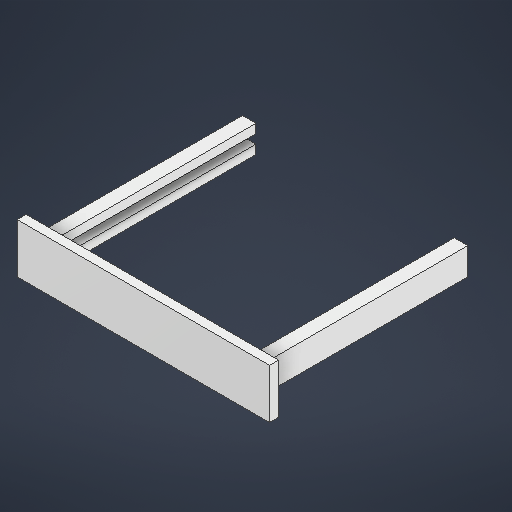
# Autodesk Inventor part: clip_pcb-command
Saved by Autodesk Inventor 2025.4 (Build 294407000, 407)
## iProperties
Created: 2025-12-22
Part Number: clip_pcb-command
Material: ABS Plastic
Document SubType Name: Modeling
Designer: sam
Density: 1.06 g/cm^3
Appearance: Smooth - White
Author: sam
Autodesk Inventor part; units mm, degrees
ref_plane "YZ Plane" through (0, 0, 0) normal (1, 0, 0) x (0, 1, 0)
ref_plane "XZ Plane" through (0, 0, 0) normal (0, 1, 0) x (-1, 0, 0)
ref_plane "XY Plane" through (0, 0, 0) normal (0, 0, 1) x (1, 0, 0)
sketch "Sketch1" plane through (0, 0, 0) normal (0, 1, 0) x (-1, 0, 0)
  line L0 (-25, -25) -> (25, -25)
  line L1 (25, -25) -> (25, 25)
  line L2 (25, 25) -> (-25, 25)
  line L3 (-25, 25) -> (-25, -25)
  line L4 (-25, -25) -> (25, 25) construction
  line L5 (25, -25) -> (-25, 25) construction
  line L6 (25, 21) -> (-25, 21)
  line L7 (22, 21) -> (22, -25)
  line L8 (-22, 21) -> (-22, -25)
  point P0 (0, 0)
  dimension "d0" = 50
  dimension "d1" = 50
  dimension "d2" = 4
  dimension "d3" = 3
  dimension "d4" = 3
  constraints: 18 end point, 6 point on line, 4 perpendicular, 2 midpoint, 2 parallel, 1 horizontal
  measures "d0" distance of L2.end L1.end
  measures "d1" distance of L1.end L0.end
  measures "d2" distance between parallel lines of L2 L6
  measures "d3" distance between parallel lines of L3 L8
  measures "d4" distance between parallel lines of L1 L7
extrude "Extrusion1" add sketch "Sketch1" along normal blind 2 contours L3 L6 L8 L0 | L3 L2 L1 L6 | L7 L6 L1 L0
sketch "Sketch2" plane through (0, 2, 0) normal (0, 1, 0) x (1, 0, 0)
  line L0 (-22, 25) -> (-25, 25) projected
  line L1 (-25, 25) -> (-25, -25) projected
  line L2 (-25, -25) -> (25, -25) projected
  line L3 (25, -25) -> (25, 25) projected
  line L4 (25, 25) -> (22, 25) projected
  line L5 (22, 25) -> (22, -21) projected
  line L6 (22, -21) -> (-22, -21) projected
  line L7 (-22, -21) -> (-22, 25) projected
  line L8 (-25, -25) -> (25, -25)
  line L9 (25, -25) -> (25, -23)
  line L10 (25, -23) -> (-25, -23)
  line L11 (-25, -23) -> (-25, -25)
  point P0 (0, 0)
  dimension "d7" = 2
  constraints: 8 end point, 2 parallel, 1 horizontal, 1 perpendicular, 1 point on line
  measures "d7" distance of L9.end L8.end
extrude "Extrusion2" add sketch "Sketch2" along normal blind 9 contours L10 L3 L2 L1
sketch "Sketch3" plane through (0, 2, 0) normal (0, 1, 0) x (1, 0, 0)
  line L0 (-25, -23) -> (25, -23) projected
  line L1 (25, -23) -> (25, 25) projected
  line L2 (25, 25) -> (22, 25) projected
  line L3 (22, 25) -> (22, -21) projected
  line L4 (22, -21) -> (-22, -21) projected
  line L5 (-22, -21) -> (-22, 25) projected
  line L6 (-22, 25) -> (-25, 25) projected
  line L7 (-25, 25) -> (-25, -23) projected
  line L8 (-25, -23) -> (-24.2, -23)
  line L9 (-24.2, -23) -> (-24.2, 25)
  line L10 (-24.2, 25) -> (-25, 25)
  line L11 (-25, 25) -> (-25, -23)
  line L12 (25, -23) -> (24.2, -23)
  line L13 (24.2, -23) -> (24.2, 25)
  line L14 (24.2, 25) -> (25, 25)
  line L15 (25, 25) -> (25, -23)
  point P0 (0, 0)
  dimension "d10" = 0.8
  dimension "d11" = 0.8
  constraints: 16 end point, 4 parallel, 2 horizontal, 2 perpendicular, 2 point on line
  measures "d10" distance of L10.end L9.end
  measures "d11" distance of L13.end L14.end
extrude "Extrusion3" add sketch "Sketch3" along normal blind 2 contours L7 L6 L9 L0 | L13 L2 L1 L0
sketch "Sketch4" plane through (0, 4, 0) normal (0, 1, 0) x (1, 0, 0)
  line L0 (-24.2, 25) -> (-25, 25) projected
  line L1 (-25, 25) -> (-25, -23) projected
  line L2 (-24.2, -23) -> (-25, -23) projected
  line L3 (-24.2, -23) -> (-24.2, 25) projected
  line L4 (24.2, -23) -> (24.2, 25) projected
  line L5 (24.2, 25) -> (22, 25) projected
  line L6 (22, 25) -> (22, -21) projected
  line L7 (22, -21) -> (-22, -21) projected
  line L8 (-22, -21) -> (-22, 25) projected
  line L9 (-22, 25) -> (-24.2, 25) projected
  line L10 (-24.2, 25) -> (-24.2, -23) projected
  line L11 (-24.2, -23) -> (24.2, -23) projected
  line L12 (-25, 25) -> (-22, 25)
  line L13 (-22, 25) -> (-22, -23)
  line L14 (-22, -23) -> (-25, -23)
  line L15 (-25, -23) -> (-25, 25)
  line L16 (25, -23) -> (24.2, -23) projected
  line L17 (25, -23) -> (25, 25) projected
  line L18 (25, 25) -> (24.2, 25) projected
  line L19 (24.2, 25) -> (24.2, -23) projected
  line L20 (25, -23) -> (22, -23)
  line L21 (22, -23) -> (22, 25)
  line L22 (22, 25) -> (25, 25)
  line L23 (25, 25) -> (25, -23)
  point P0 (0, 0)
  constraints: 16 end point, 4 parallel, 2 horizontal, 2 perpendicular, 1 point on line
extrude "Extrusion4" add sketch "Sketch4" along normal blind 2 contours L3 L2 L1 L0 | L9 L8 L13 L11 L3 | L21 L6 L5 L4 L11 | L4 L18 L17 L16
sketch "Sketch5" plane through (25, 0, 25) normal (1, 0, 0) x (0, 0, -1)
  line L0 (0, 11) -> (2, 11) projected
  line L1 (0, 0) -> (0, 11) projected
  line L2 (2, 11) -> (0, 11)
  line L3 (0, 11) -> (0, 0)
  line L4 (0, 0) -> (2, 0)
  line L5 (2, 0) -> (2, 11)
  point P0 (25, 0)
  constraints: 8 end point, 2 parallel, 1 horizontal, 1 perpendicular
extrude "Extrusion5" add sketch "Sketch5" along normal blind 6
body "Solid1"
